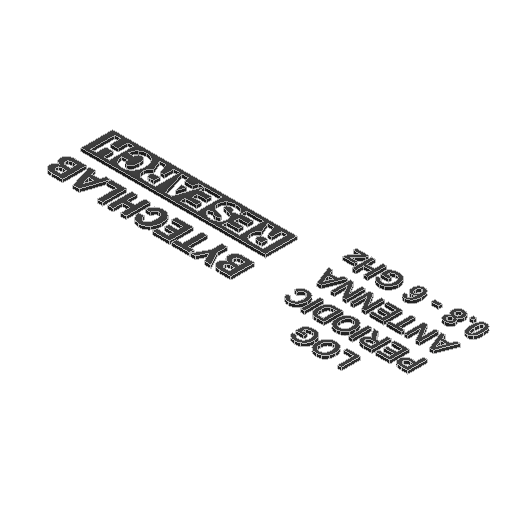
# Autodesk Inventor part: 3DP_PLA_Antenna_Case_Top_Logo_and_Name
Saved by Autodesk Inventor 2026.1 (Build 301233000, 233)
## iProperties
Created: 2025-11-20
Part Number: 3DP_PLA_Antenna_Case_Top_Logo_and_Name
Material: Generic
Document SubType Name: Modeling
Designer: User
Density: 1 g/cm^3
Appearance: Rubber - Black
Author: User
Autodesk Inventor part; units mm, degrees
(part 1 of 2)
ref_plane "YZ Plane" through (0, 0, 0) normal (1, 0, 0) x (0, 1, 0)
ref_plane "XZ Plane" through (0, 0, 0) normal (0, 1, 0) x (-1, 0, 0)
ref_plane "XY Plane" through (0, 0, 0) normal (0, 0, 1) x (1, 0, 0)
sketch "Sketch1" plane through (0, 0, 0) normal (0, 1, 0) x (-1, 0, 0)
  spline S0 degree 3 poles (1.4594, 11.82) (2.0835, 11.82) (2.5525, 11.7433) (2.8664, 11.59) knots 0 0 0 0 1 1 1 1
  line L0 (1.4594, 11.82) -> (2.0835, 11.82) construction
  line L1 (2.0835, 11.82) -> (2.5525, 11.7433) construction
  line L2 (2.5525, 11.7433) -> (2.8664, 11.59) construction
  spline S1 degree 3 poles (2.8664, 11.59) (3.1803, 11.4367) (3.4394, 11.2177) (3.6438, 10.933) knots 0 0 0 0 1 1 1 1
  line L3 (2.8664, 11.59) -> (3.1803, 11.4367) construction
  line L4 (3.1803, 11.4367) -> (3.4394, 11.2177) construction
  line L5 (3.4394, 11.2177) -> (3.6438, 10.933) construction
  spline S2 degree 3 poles (3.6438, 10.933) (3.8482, 10.6483) (3.9504, 10.3016) (3.9504, 9.8928) knots 0 0 0 0 1 1 1 1
  line L6 (3.6438, 10.933) -> (3.8482, 10.6483) construction
  line L7 (3.8482, 10.6483) -> (3.9504, 10.3016) construction
  line L8 (3.9504, 10.3016) -> (3.9504, 9.8928) construction
  spline S3 degree 3 poles (3.9504, 9.8928) (3.9504, 9.0643) (3.5015, 8.5113) (2.6036, 8.2339) knots 0 0 0 0 1 1 1 1
  line L9 (3.9504, 9.8928) -> (3.9504, 9.0643) construction
  line L10 (3.9504, 9.0643) -> (3.5015, 8.5113) construction
  line L11 (3.5015, 8.5113) -> (2.6036, 8.2339) construction
  spline S4 degree 3 poles (2.6036, 8.2339) (3.1219, 8.1171) (3.5106, 7.8854) (3.7698, 7.5386) knots 0 0 0 0 1 1 1 1
  line L12 (2.6036, 8.2339) -> (3.1219, 8.1171) construction
  line L13 (3.1219, 8.1171) -> (3.5106, 7.8854) construction
  line L14 (3.5106, 7.8854) -> (3.7698, 7.5386) construction
  spline S5 degree 3 poles (3.7698, 7.5386) (4.0289, 7.1919) (4.1585, 6.8141) (4.1585, 6.4053) knots 0 0 0 0 1 1 1 1
  line L15 (3.7698, 7.5386) -> (4.0289, 7.1919) construction
  line L16 (4.0289, 7.1919) -> (4.1585, 6.8141) construction
  line L17 (4.1585, 6.8141) -> (4.1585, 6.4053) construction
  spline S6 degree 3 poles (4.1585, 6.4053) (4.1585, 5.8469) (3.9468, 5.3633) (3.5234, 4.9545) knots 0 0 0 0 1 1 1 1
  line L18 (4.1585, 6.4053) -> (4.1585, 5.8469) construction
  line L19 (4.1585, 5.8469) -> (3.9468, 5.3633) construction
  line L20 (3.9468, 5.3633) -> (3.5234, 4.9545) construction
  spline S7 degree 3 poles (3.5234, 4.9545) (3.1, 4.5494) (2.412, 4.3468) (1.4594, 4.3468) knots 0 0 0 0 1 1 1 1
  line L21 (3.5234, 4.9545) -> (3.1, 4.5494) construction
  line L22 (3.1, 4.5494) -> (2.412, 4.3468) construction
  line L23 (2.412, 4.3468) -> (1.4594, 4.3468) construction
  line L24 (-2.0226, 11.82) -> (1.4594, 11.82)
  line L25 (1.4594, 4.3468) -> (-2.0226, 4.3468)
  line L26 (-2.0226, 4.3468) -> (-2.0226, 11.82)
  spline S8 degree 3 poles (1.0488, 8.8635) (1.5342, 8.8635) (1.839, 8.9584) (1.9631, 9.1482) knots 0 0 0 0 1 1 1 1
  line L27 (1.0488, 8.8635) -> (1.5342, 8.8635) construction
  line L28 (1.5342, 8.8635) -> (1.839, 8.9584) construction
  line L29 (1.839, 8.9584) -> (1.9631, 9.1482) construction
  spline S9 degree 3 poles (1.9631, 9.1482) (2.0908, 9.3417) (2.1547, 9.526) (2.1547, 9.7012) knots 0 0 0 0 1 1 1 1
  line L30 (1.9631, 9.1482) -> (2.0908, 9.3417) construction
  line L31 (2.0908, 9.3417) -> (2.1547, 9.526) construction
  line L32 (2.1547, 9.526) -> (2.1547, 9.7012) construction
  spline S10 degree 3 poles (2.1547, 9.7012) (2.1547, 9.891) (2.1017, 10.0534) (1.9959, 10.1885) knots 0 0 0 0 1 1 1 1
  line L33 (2.1547, 9.7012) -> (2.1547, 9.891) construction
  line L34 (2.1547, 9.891) -> (2.1017, 10.0534) construction
  line L35 (2.1017, 10.0534) -> (1.9959, 10.1885) construction
  spline S11 degree 3 poles (1.9959, 10.1885) (1.8937, 10.3272) (1.7806, 10.4129) (1.6565, 10.4458) knots 0 0 0 0 1 1 1 1
  line L36 (1.9959, 10.1885) -> (1.8937, 10.3272) construction
  line L37 (1.8937, 10.3272) -> (1.7806, 10.4129) construction
  line L38 (1.7806, 10.4129) -> (1.6565, 10.4458) construction
  spline S12 degree 3 poles (1.6565, 10.4458) (1.5324, 10.4823) (1.2878, 10.5005) (0.9228, 10.5005) knots 0 0 0 0 1 1 1 1
  line L39 (1.6565, 10.4458) -> (1.5324, 10.4823) construction
  line L40 (1.5324, 10.4823) -> (1.2878, 10.5005) construction
  line L41 (1.2878, 10.5005) -> (0.9228, 10.5005) construction
  line L42 (-0.2762, 10.5005) -> (-0.2762, 8.8635)
  line L43 (-0.2762, 8.8635) -> (1.0488, 8.8635)
  line L44 (0.9228, 10.5005) -> (-0.2762, 10.5005)
  spline S13 degree 3 poles (1.0707, 5.7319) (1.5305, 5.7319) (1.8554, 5.8122) (2.0452, 5.9728) knots 0 0 0 0 1 1 1 1
  line L45 (1.0707, 5.7319) -> (1.5305, 5.7319) construction
  line L46 (1.5305, 5.7319) -> (1.8554, 5.8122) construction
  line L47 (1.8554, 5.8122) -> (2.0452, 5.9728) construction
  spline S14 degree 3 poles (2.0452, 5.9728) (2.235, 6.1334) (2.3299, 6.3579) (2.3299, 6.6462) knots 0 0 0 0 1 1 1 1
  line L48 (2.0452, 5.9728) -> (2.235, 6.1334) construction
  line L49 (2.235, 6.1334) -> (2.3299, 6.3579) construction
  line L50 (2.3299, 6.3579) -> (2.3299, 6.6462) construction
  spline S15 degree 3 poles (2.3299, 6.6462) (2.3299, 6.8871) (2.2386, 7.0952) (2.0561, 7.2704) knots 0 0 0 0 1 1 1 1
  line L51 (2.3299, 6.6462) -> (2.3299, 6.8871) construction
  line L52 (2.3299, 6.8871) -> (2.2386, 7.0952) construction
  line L53 (2.2386, 7.0952) -> (2.0561, 7.2704) construction
  spline S16 degree 3 poles (2.0561, 7.2704) (1.8736, 7.4456) (1.5707, 7.5332) (1.1473, 7.5332) knots 0 0 0 0 1 1 1 1
  line L54 (2.0561, 7.2704) -> (1.8736, 7.4456) construction
  line L55 (1.8736, 7.4456) -> (1.5707, 7.5332) construction
  line L56 (1.5707, 7.5332) -> (1.1473, 7.5332) construction
  line L57 (-0.2762, 7.5332) -> (-0.2762, 5.7319)
  line L58 (-0.2762, 5.7319) -> (1.0707, 5.7319)
  line L59 (1.1473, 7.5332) -> (-0.2762, 7.5332)
  line L60 (10.5805, 11.82) -> (8.2318, 7.4948)
  line L61 (8.2318, 7.4948) -> (8.2318, 4.3468)
  line L62 (8.2318, 4.3468) -> (6.4798, 4.3468)
  line L63 (6.4798, 4.3468) -> (6.4798, 7.4948)
  line L64 (6.4798, 7.4948) -> (4.1311, 11.82)
  line L65 (4.1311, 11.82) -> (6.1623, 11.82)
  line L66 (6.1623, 11.82) -> (7.5912, 8.984)
  line L67 (7.5912, 8.984) -> (9.0092, 11.82)
  line L68 (9.0092, 11.82) -> (10.5805, 11.82)
  line L69 (16.2907, 11.82) -> (16.2907, 10.3418)
  line L70 (16.2907, 10.3418) -> (14.4402, 10.3418)
  line L71 (14.4402, 10.3418) -> (14.4402, 4.3468)
  line L72 (14.4402, 4.3468) -> (12.6664, 4.3468)
  line L73 (12.6664, 4.3468) -> (12.6664, 10.3418)
  line L74 (12.6664, 10.3418) -> (10.8049, 10.3418)
  line L75 (10.8049, 10.3418) -> (10.8049, 11.82)
  line L76 (10.8049, 11.82) -> (16.2907, 11.82)
  line L77 (22.3788, 10.3965) -> (18.8147, 10.3965)
  line L78 (18.8147, 10.3965) -> (18.8147, 8.8635)
  line L79 (18.8147, 8.8635) -> (21.6178, 8.8635)
  line L80 (21.6178, 8.8635) -> (21.6178, 7.4565)
  line L81 (21.6178, 7.4565) -> (18.8147, 7.4565)
  line L82 (18.8147, 7.4565) -> (18.8147, 5.825)
  line L83 (18.8147, 5.825) -> (22.3788, 5.825)
  line L84 (22.3788, 5.825) -> (22.3788, 4.3468)
  line L85 (22.3788, 4.3468) -> (17.0353, 4.3468)
  line L86 (17.0353, 4.3468) -> (17.0353, 11.82)
  line L87 (17.0353, 11.82) -> (22.3788, 11.82)
  line L88 (22.3788, 11.82) -> (22.3788, 10.3965)
  spline S17 degree 3 poles (27.6237, 8.9238) (27.5981, 9.9786) (27.1875, 10.506) (26.3919, 10.506) knots 0 0 0 0 1 1 1 1
  line L89 (27.6237, 8.9238) -> (27.5981, 9.9786) construction
  line L90 (27.5981, 9.9786) -> (27.1875, 10.506) construction
  line L91 (27.1875, 10.506) -> (26.3919, 10.506) construction
  spline S18 degree 3 poles (26.3919, 10.506) (25.4794, 10.506) (25.0231, 9.6939) (25.0231, 8.0697) knots 0 0 0 0 1 1 1 1
  line L92 (26.3919, 10.506) -> (25.4794, 10.506) construction
  line L93 (25.4794, 10.506) -> (25.0231, 9.6939) construction
  line L94 (25.0231, 9.6939) -> (25.0231, 8.0697) construction
  spline S19 degree 3 poles (25.0231, 8.0697) (25.0231, 7.1317) (25.1472, 6.4948) (25.3954, 6.159) knots 0 0 0 0 1 1 1 1
  line L95 (25.0231, 8.0697) -> (25.0231, 7.1317) construction
  line L96 (25.0231, 7.1317) -> (25.1472, 6.4948) construction
  line L97 (25.1472, 6.4948) -> (25.3954, 6.159) construction
  spline S20 degree 3 poles (25.3954, 6.159) (25.6436, 5.8268) (25.9904, 5.6608) (26.4357, 5.6608) knots 0 0 0 0 1 1 1 1
  line L98 (25.3954, 6.159) -> (25.6436, 5.8268) construction
  line L99 (25.6436, 5.8268) -> (25.9904, 5.6608) construction
  line L100 (25.9904, 5.6608) -> (26.4357, 5.6608) construction
  spline S21 degree 3 poles (26.4357, 5.6608) (27.1583, 5.6608) (27.6, 6.1316) (27.7606, 7.0733) knots 0 0 0 0 1 1 1 1
  line L101 (26.4357, 5.6608) -> (27.1583, 5.6608) construction
  line L102 (27.1583, 5.6608) -> (27.6, 6.1316) construction
  line L103 (27.6, 6.1316) -> (27.7606, 7.0733) construction
  line L104 (29.4578, 9.0387) -> (27.6237, 8.9238)
  spline S22 degree 3 poles (29.4578, 6.9692) (29.3483, 6.075) (29.0143, 5.3943) (28.4559, 4.9271) knots 0 0 0 0 1 1 1 1
  line L105 (29.4578, 6.9692) -> (29.3483, 6.075) construction
  line L106 (29.3483, 6.075) -> (29.0143, 5.3943) construction
  line L107 (29.0143, 5.3943) -> (28.4559, 4.9271) construction
  spline S23 degree 3 poles (28.4559, 4.9271) (27.9011, 4.4636) (27.2204, 4.2318) (26.4138, 4.2318) knots 0 0 0 0 1 1 1 1
  line L108 (28.4559, 4.9271) -> (27.9011, 4.4636) construction
  line L109 (27.9011, 4.4636) -> (27.2204, 4.2318) construction
  line L110 (27.2204, 4.2318) -> (26.4138, 4.2318) construction
  spline S24 degree 3 poles (26.4138, 4.2318) (25.4246, 4.2318) (24.6198, 4.5731) (23.9993, 5.2556) knots 0 0 0 0 1 1 1 1
  line L111 (26.4138, 4.2318) -> (25.4246, 4.2318) construction
  line L112 (25.4246, 4.2318) -> (24.6198, 4.5731) construction
  line L113 (24.6198, 4.5731) -> (23.9993, 5.2556) construction
  spline S25 degree 3 poles (23.9993, 5.2556) (23.3825, 5.9381) (23.0741, 6.8816) (23.0741, 8.0861) knots 0 0 0 0 1 1 1 1
  line L114 (23.9993, 5.2556) -> (23.3825, 5.9381) construction
  line L115 (23.3825, 5.9381) -> (23.0741, 6.8816) construction
  line L116 (23.0741, 6.8816) -> (23.0741, 8.0861) construction
  spline S26 degree 3 poles (23.0741, 8.0861) (23.0741, 9.2139) (23.3734, 10.1374) (23.972, 10.8564) knots 0 0 0 0 1 1 1 1
  line L117 (23.0741, 8.0861) -> (23.0741, 9.2139) construction
  line L118 (23.0741, 9.2139) -> (23.3734, 10.1374) construction
  line L119 (23.3734, 10.1374) -> (23.972, 10.8564) construction
  spline S27 degree 3 poles (23.972, 10.8564) (24.5706, 11.5754) (25.3881, 11.9349) (26.4247, 11.9349) knots 0 0 0 0 1 1 1 1
  line L120 (23.972, 10.8564) -> (24.5706, 11.5754) construction
  line L121 (24.5706, 11.5754) -> (25.3881, 11.9349) construction
  line L122 (25.3881, 11.9349) -> (26.4247, 11.9349) construction
  spline S28 degree 3 poles (26.4247, 11.9349) (28.2205, 11.9349) (29.2315, 10.9695) (29.4578, 9.0387) knots 0 0 0 0 1 1 1 1
  line L123 (26.4247, 11.9349) -> (28.2205, 11.9349) construction
  line L124 (28.2205, 11.9349) -> (29.2315, 10.9695) construction
  line L125 (29.2315, 10.9695) -> (29.4578, 9.0387) construction
  line L126 (27.7606, 7.0733) -> (29.4578, 6.9692)
  line L127 (36.2411, 11.82) -> (36.2411, 4.3468)
  line L128 (36.2411, 4.3468) -> (34.522, 4.3468)
  line L129 (34.522, 4.3468) -> (34.522, 7.4291)
  line L130 (34.522, 7.4291) -> (32.1843, 7.4291)
  line L131 (32.1843, 7.4291) -> (32.1843, 4.3468)
  line L132 (32.1843, 4.3468) -> (30.4651, 4.3468)
  line L133 (30.4651, 4.3468) -> (30.4651, 11.82)
  line L134 (30.4651, 11.82) -> (32.1843, 11.82)
  line L135 (32.1843, 11.82) -> (32.1843, 8.9073)
  line L136 (32.1843, 8.9073) -> (34.522, 8.9073)
  line L137 (34.522, 8.9073) -> (34.522, 11.82)
  line L138 (34.522, 11.82) -> (36.2411, 11.82)
  line L139 (39.5096, 5.825) -> (42.4824, 5.825)
  line L140 (42.4824, 5.825) -> (42.4824, 4.3468)
  line L141 (42.4824, 4.3468) -> (37.7358, 4.3468)
  line L142 (37.7358, 4.3468) -> (37.7358, 11.82)
  line L143 (37.7358, 11.82) -> (39.5096, 11.82)
  line L144 (39.5096, 11.82) -> (39.5096, 5.825)
  line L145 (47.054, 11.82) -> (49.3917, 4.3468)
  line L146 (49.3917, 4.3468) -> (47.5084, 4.3468)
  line L147 (47.5084, 4.3468) -> (47.054, 5.8852)
  line L148 (47.054, 5.8852) -> (44.6341, 5.8852)
  line L149 (44.6341, 5.8852) -> (44.1632, 4.3468)
  line L150 (44.1632, 4.3468) -> (42.6303, 4.3468)
  line L151 (42.6303, 4.3468) -> (45.0228, 11.82)
  line L152 (45.0228, 11.82) -> (47.054, 11.82)
  line L153 (45.0556, 7.2649) -> (46.6433, 7.2649)
  line L154 (46.6433, 7.2649) -> (45.8495, 9.8873)
  line L155 (45.8495, 9.8873) -> (45.0556, 7.2649)
  spline S29 degree 3 poles (53.6785, 11.82) (54.3027, 11.82) (54.7717, 11.7433) (55.0856, 11.59) knots 0 0 0 0 1 1 1 1
  line L156 (53.6785, 11.82) -> (54.3027, 11.82) construction
  line L157 (54.3027, 11.82) -> (54.7717, 11.7433) construction
  line L158 (54.7717, 11.7433) -> (55.0856, 11.59) construction
  spline S30 degree 3 poles (55.0856, 11.59) (55.3995, 11.4367) (55.6586, 11.2177) (55.863, 10.933) knots 0 0 0 0 1 1 1 1
  line L159 (55.0856, 11.59) -> (55.3995, 11.4367) construction
  line L160 (55.3995, 11.4367) -> (55.6586, 11.2177) construction
  line L161 (55.6586, 11.2177) -> (55.863, 10.933) construction
  spline S31 degree 3 poles (55.863, 10.933) (56.0674, 10.6483) (56.1696, 10.3016) (56.1696, 9.8928) knots 0 0 0 0 1 1 1 1
  line L162 (55.863, 10.933) -> (56.0674, 10.6483) construction
  line L163 (56.0674, 10.6483) -> (56.1696, 10.3016) construction
  line L164 (56.1696, 10.3016) -> (56.1696, 9.8928) construction
  spline S32 degree 3 poles (56.1696, 9.8928) (56.1696, 9.0643) (55.7206, 8.5113) (54.8228, 8.2339) knots 0 0 0 0 1 1 1 1
  line L165 (56.1696, 9.8928) -> (56.1696, 9.0643) construction
  line L166 (56.1696, 9.0643) -> (55.7206, 8.5113) construction
  line L167 (55.7206, 8.5113) -> (54.8228, 8.2339) construction
  spline S33 degree 3 poles (54.8228, 8.2339) (55.3411, 8.1171) (55.7298, 7.8854) (55.9889, 7.5386) knots 0 0 0 0 1 1 1 1
  line L168 (54.8228, 8.2339) -> (55.3411, 8.1171) construction
  line L169 (55.3411, 8.1171) -> (55.7298, 7.8854) construction
  line L170 (55.7298, 7.8854) -> (55.9889, 7.5386) construction
  spline S34 degree 3 poles (55.9889, 7.5386) (56.2481, 7.1919) (56.3776, 6.8141) (56.3776, 6.4053) knots 0 0 0 0 1 1 1 1
  line L171 (55.9889, 7.5386) -> (56.2481, 7.1919) construction
  line L172 (56.2481, 7.1919) -> (56.3776, 6.8141) construction
  line L173 (56.3776, 6.8141) -> (56.3776, 6.4053) construction
  spline S35 degree 3 poles (56.3776, 6.4053) (56.3776, 5.8469) (56.1659, 5.3633) (55.7425, 4.9545) knots 0 0 0 0 1 1 1 1
  line L174 (56.3776, 6.4053) -> (56.3776, 5.8469) construction
  line L175 (56.3776, 5.8469) -> (56.1659, 5.3633) construction
  line L176 (56.1659, 5.3633) -> (55.7425, 4.9545) construction
  spline S36 degree 3 poles (55.7425, 4.9545) (55.3192, 4.5494) (54.6312, 4.3468) (53.6785, 4.3468) knots 0 0 0 0 1 1 1 1
  line L177 (55.7425, 4.9545) -> (55.3192, 4.5494) construction
  line L178 (55.3192, 4.5494) -> (54.6312, 4.3468) construction
  line L179 (54.6312, 4.3468) -> (53.6785, 4.3468) construction
  line L180 (50.1965, 11.82) -> (53.6785, 11.82)
  line L181 (53.6785, 4.3468) -> (50.1965, 4.3468)
  line L182 (50.1965, 4.3468) -> (50.1965, 11.82)
  spline S37 degree 3 poles (53.2679, 8.8635) (53.7534, 8.8635) (54.0581, 8.9584) (54.1822, 9.1482) knots 0 0 0 0 1 1 1 1
  line L183 (53.2679, 8.8635) -> (53.7534, 8.8635) construction
  line L184 (53.7534, 8.8635) -> (54.0581, 8.9584) construction
  line L185 (54.0581, 8.9584) -> (54.1822, 9.1482) construction
  spline S38 degree 3 poles (54.1822, 9.1482) (54.31, 9.3417) (54.3738, 9.526) (54.3738, 9.7012) knots 0 0 0 0 1 1 1 1
  line L186 (54.1822, 9.1482) -> (54.31, 9.3417) construction
  line L187 (54.31, 9.3417) -> (54.3738, 9.526) construction
  line L188 (54.3738, 9.526) -> (54.3738, 9.7012) construction
  spline S39 degree 3 poles (54.3738, 9.7012) (54.3738, 9.891) (54.3209, 10.0534) (54.2151, 10.1885) knots 0 0 0 0 1 1 1 1
  line L189 (54.3738, 9.7012) -> (54.3738, 9.891) construction
  line L190 (54.3738, 9.891) -> (54.3209, 10.0534) construction
  line L191 (54.3209, 10.0534) -> (54.2151, 10.1885) construction
  spline S40 degree 3 poles (54.2151, 10.1885) (54.1129, 10.3272) (53.9997, 10.4129) (53.8756, 10.4458) knots 0 0 0 0 1 1 1 1
  line L192 (54.2151, 10.1885) -> (54.1129, 10.3272) construction
  line L193 (54.1129, 10.3272) -> (53.9997, 10.4129) construction
  line L194 (53.9997, 10.4129) -> (53.8756, 10.4458) construction
  spline S41 degree 3 poles (53.8756, 10.4458) (53.7515, 10.4823) (53.507, 10.5005) (53.142, 10.5005) knots 0 0 0 0 1 1 1 1
  line L195 (53.8756, 10.4458) -> (53.7515, 10.4823) construction
  line L196 (53.7515, 10.4823) -> (53.507, 10.5005) construction
  line L197 (53.507, 10.5005) -> (53.142, 10.5005) construction
  line L198 (51.943, 10.5005) -> (51.943, 8.8635)
  line L199 (51.943, 8.8635) -> (53.2679, 8.8635)
  line L200 (53.142, 10.5005) -> (51.943, 10.5005)
  spline S42 degree 3 poles (53.2898, 5.7319) (53.7497, 5.7319) (54.0745, 5.8122) (54.2643, 5.9728) knots 0 0 0 0 1 1 1 1
  line L201 (53.2898, 5.7319) -> (53.7497, 5.7319) construction
  line L202 (53.7497, 5.7319) -> (54.0745, 5.8122) construction
  line L203 (54.0745, 5.8122) -> (54.2643, 5.9728) construction
  spline S43 degree 3 poles (54.2643, 5.9728) (54.4541, 6.1334) (54.549, 6.3579) (54.549, 6.6462) knots 0 0 0 0 1 1 1 1
  line L204 (54.2643, 5.9728) -> (54.4541, 6.1334) construction
  line L205 (54.4541, 6.1334) -> (54.549, 6.3579) construction
  line L206 (54.549, 6.3579) -> (54.549, 6.6462) construction
  spline S44 degree 3 poles (54.549, 6.6462) (54.549, 6.8871) (54.4578, 7.0952) (54.2753, 7.2704) knots 0 0 0 0 1 1 1 1
  line L207 (54.549, 6.6462) -> (54.549, 6.8871) construction
  line L208 (54.549, 6.8871) -> (54.4578, 7.0952) construction
  line L209 (54.4578, 7.0952) -> (54.2753, 7.2704) construction
  spline S45 degree 3 poles (54.2753, 7.2704) (54.0928, 7.4456) (53.7898, 7.5332) (53.3665, 7.5332) knots 0 0 0 0 1 1 1 1
  line L210 (54.2753, 7.2704) -> (54.0928, 7.4456) construction
  line L211 (54.0928, 7.4456) -> (53.7898, 7.5332) construction
  line L212 (53.7898, 7.5332) -> (53.3665, 7.5332) construction
  line L213 (51.943, 7.5332) -> (51.943, 5.7319)
  line L214 (51.943, 5.7319) -> (53.2898, 5.7319)
  line L215 (53.3665, 7.5332) -> (51.943, 7.5332)
  line L216 (-1.4592, 0.5085) -> (55.8142, 0.5085)
  line L217 (55.8142, 0.5085) -> (55.8142, -9.3243)
  line L218 (55.8142, -9.3243) -> (-1.4592, -9.3243)
  line L219 (-1.4592, -9.3243) -> (-1.4592, 0.5085)
  spline S46 degree 3 poles (3.7095, -0.6713) (4.3154, -0.6713) (4.8009, -0.7425) (5.1658, -0.8848) knots 0 0 0 0 1 1 1 1
  line L220 (3.7095, -0.6713) -> (4.3154, -0.6713) construction
  line L221 (4.3154, -0.6713) -> (4.8009, -0.7425) construction
  line L222 (4.8009, -0.7425) -> (5.1658, -0.8848) construction
  spline S47 degree 3 poles (5.1658, -0.8848) (5.5345, -1.0235) (5.8393, -1.2808) (6.0801, -1.6568) knots 0 0 0 0 1 1 1 1
  line L223 (5.1658, -0.8848) -> (5.5345, -1.0235) construction
  line L224 (5.5345, -1.0235) -> (5.8393, -1.2808) construction
  line L225 (5.8393, -1.2808) -> (6.0801, -1.6568) construction
  spline S48 degree 3 poles (6.0801, -1.6568) (6.321, -2.0327) (6.4415, -2.4506) (6.4415, -2.9105) knots 0 0 0 0 1 1 1 1
  line L226 (6.0801, -1.6568) -> (6.321, -2.0327) construction
  line L227 (6.321, -2.0327) -> (6.4415, -2.4506) construction
  line L228 (6.4415, -2.4506) -> (6.4415, -2.9105) construction
  spline S49 degree 3 poles (6.4415, -2.9105) (6.4415, -3.8084) (6.009, -4.4526) (5.1439, -4.8431) knots 0 0 0 0 1 1 1 1
  line L229 (6.4415, -2.9105) -> (6.4415, -3.8084) construction
  line L230 (6.4415, -3.8084) -> (6.009, -4.4526) construction
  line L231 (6.009, -4.4526) -> (5.1439, -4.8431) construction
  line L232 (2.1875, -5.1826) -> (2.1875, -8.1445)
  line L233 (2.1875, -8.1445) -> (0.4246, -8.1445)
  line L234 (0.4246, -8.1445) -> (0.4246, -0.6713)
  line L235 (0.4246, -0.6713) -> (3.7095, -0.6713)
  line L236 (5.1439, -4.8431) -> (6.5236, -8.1445)
  line L237 (6.5236, -8.1445) -> (4.591, -8.1445)
  line L238 (4.591, -8.1445) -> (3.4413, -5.1826)
  line L239 (3.4413, -5.1826) -> (2.1875, -5.1826)
  spline S50 degree 3 poles (3.2606, -3.9069) (3.611, -3.9069) (3.8647, -3.8832) (4.0216, -3.8358) knots 0 0 0 0 1 1 1 1
  line L240 (3.2606, -3.9069) -> (3.611, -3.9069) construction
  line L241 (3.611, -3.9069) -> (3.8647, -3.8832) construction
  line L242 (3.8647, -3.8832) -> (4.0216, -3.8358) construction
  spline S51 degree 3 poles (4.0216, -3.8358) (4.1822, -3.7847) (4.3245, -3.6752) (4.4486, -3.5073) knots 0 0 0 0 1 1 1 1
  line L243 (4.0216, -3.8358) -> (4.1822, -3.7847) construction
  line L244 (4.1822, -3.7847) -> (4.3245, -3.6752) construction
  line L245 (4.3245, -3.6752) -> (4.4486, -3.5073) construction
  spline S52 degree 3 poles (4.4486, -3.5073) (4.5727, -3.3357) (4.6348, -3.1405) (4.6348, -2.9215) knots 0 0 0 0 1 1 1 1
  line L246 (4.4486, -3.5073) -> (4.5727, -3.3357) construction
  line L247 (4.5727, -3.3357) -> (4.6348, -3.1405) construction
  line L248 (4.6348, -3.1405) -> (4.6348, -2.9215) construction
  spline S53 degree 3 poles (4.6348, -2.9215) (4.6348, -2.7134) (4.5727, -2.5273) (4.4486, -2.363) knots 0 0 0 0 1 1 1 1
  line L249 (4.6348, -2.9215) -> (4.6348, -2.7134) construction
  line L250 (4.6348, -2.7134) -> (4.5727, -2.5273) construction
  line L251 (4.5727, -2.5273) -> (4.4486, -2.363) construction
  spline S54 degree 3 poles (4.4486, -2.363) (4.3245, -2.1988) (4.1895, -2.0984) (4.0435, -2.0619) knots 0 0 0 0 1 1 1 1
  line L252 (4.4486, -2.363) -> (4.3245, -2.1988) construction
  line L253 (4.3245, -2.1988) -> (4.1895, -2.0984) construction
  line L254 (4.1895, -2.0984) -> (4.0435, -2.0619) construction
  spline S55 degree 3 poles (4.0435, -2.0619) (3.8975, -2.0218) (3.6238, -2.0017) (3.2223, -2.0017) knots 0 0 0 0 1 1 1 1
  line L255 (4.0435, -2.0619) -> (3.8975, -2.0218) construction
  line L256 (3.8975, -2.0218) -> (3.6238, -2.0017) construction
  line L257 (3.6238, -2.0017) -> (3.2223, -2.0017) construction
  line L258 (2.1875, -2.0017) -> (2.1875, -3.9069)
  line L259 (2.1875, -3.9069) -> (3.2606, -3.9069)
  line L260 (3.2223, -2.0017) -> (2.1875, -2.0017)
  line L261 (13.1318, -2.0948) -> (9.5676, -2.0948)
  line L262 (9.5676, -2.0948) -> (9.5676, -3.6277)
  line L263 (9.5676, -3.6277) -> (12.3708, -3.6277)
  line L264 (12.3708, -3.6277) -> (12.3708, -5.0348)
  line L265 (12.3708, -5.0348) -> (9.5676, -5.0348)
  line L266 (9.5676, -5.0348) -> (9.5676, -6.6663)
  line L267 (9.5676, -6.6663) -> (13.1318, -6.6663)
  line L268 (13.1318, -6.6663) -> (13.1318, -8.1445)
  line L269 (13.1318, -8.1445) -> (7.7883, -8.1445)
  line L270 (7.7883, -8.1445) -> (7.7883, -0.6713)
  line L271 (7.7883, -0.6713) -> (13.1318, -0.6713)
  line L272 (13.1318, -0.6713) -> (13.1318, -2.0948)
  spline S56 degree 3 poles (17.8566, -2.812) (17.6558, -2.2207) (17.2306, -1.925) (16.5809, -1.925) knots 0 0 0 0 1 1 1 1
  line L273 (17.8566, -2.812) -> (17.6558, -2.2207) construction
  line L274 (17.6558, -2.2207) -> (17.2306, -1.925) construction
  line L275 (17.2306, -1.925) -> (16.5809, -1.925) construction
  spline S57 degree 3 poles (16.5809, -1.925) (15.8874, -1.925) (15.5407, -2.1495) (15.5407, -2.5984) knots 0 0 0 0 1 1 1 1
  line L276 (16.5809, -1.925) -> (15.8874, -1.925) construction
  line L277 (15.8874, -1.925) -> (15.5407, -2.1495) construction
  line L278 (15.5407, -2.1495) -> (15.5407, -2.5984) construction
  spline S58 degree 3 poles (15.5407, -2.5984) (15.5407, -2.7773) (15.6046, -2.9288) (15.7323, -3.0529) knots 0 0 0 0 1 1 1 1
  line L279 (15.5407, -2.5984) -> (15.5407, -2.7773) construction
  line L280 (15.5407, -2.7773) -> (15.6046, -2.9288) construction
  line L281 (15.6046, -2.9288) -> (15.7323, -3.0529) construction
  spline S59 degree 3 poles (15.7323, -3.0529) (15.8637, -3.177) (16.1575, -3.2846) (16.6138, -3.3759) knots 0 0 0 0 1 1 1 1
  line L282 (15.7323, -3.0529) -> (15.8637, -3.177) construction
  line L283 (15.8637, -3.177) -> (16.1575, -3.2846) construction
  line L284 (16.1575, -3.2846) -> (16.6138, -3.3759) construction
  spline S60 degree 3 poles (16.6138, -3.3759) (17.3766, -3.5292) (17.935, -3.6843) (18.2891, -3.8412) knots 0 0 0 0 1 1 1 1
  line L285 (16.6138, -3.3759) -> (17.3766, -3.5292) construction
  line L286 (17.3766, -3.5292) -> (17.935, -3.6843) construction
  line L287 (17.935, -3.6843) -> (18.2891, -3.8412) construction
  spline S61 degree 3 poles (18.2891, -3.8412) (18.6431, -3.9982) (18.9406, -4.2518) (19.1815, -4.6022) knots 0 0 0 0 1 1 1 1
  line L288 (18.2891, -3.8412) -> (18.6431, -3.9982) construction
  line L289 (18.6431, -3.9982) -> (18.9406, -4.2518) construction
  line L290 (18.9406, -4.2518) -> (19.1815, -4.6022) construction
  spline S62 degree 3 poles (19.1815, -4.6022) (19.426, -4.949) (19.5483, -5.3377) (19.5483, -5.7684) knots 0 0 0 0 1 1 1 1
  line L291 (19.1815, -4.6022) -> (19.426, -4.949) construction
  line L292 (19.426, -4.949) -> (19.5483, -5.3377) construction
  line L293 (19.5483, -5.3377) -> (19.5483, -5.7684) construction
  spline S63 degree 3 poles (19.5483, -5.7684) (19.5483, -6.4436) (19.2873, -7.0276) (18.7654, -7.5203) knots 0 0 0 0 1 1 1 1
  line L294 (19.5483, -5.7684) -> (19.5483, -6.4436) construction
  line L295 (19.5483, -6.4436) -> (19.2873, -7.0276) construction
  line L296 (19.2873, -7.0276) -> (18.7654, -7.5203) construction
  spline S64 degree 3 poles (18.7654, -7.5203) (18.2471, -8.0131) (17.477, -8.2594) (16.455, -8.2594) knots 0 0 0 0 1 1 1 1
  line L297 (18.7654, -7.5203) -> (18.2471, -8.0131) construction
  line L298 (18.2471, -8.0131) -> (17.477, -8.2594) construction
  line L299 (17.477, -8.2594) -> (16.455, -8.2594) construction
  spline S65 degree 3 poles (16.455, -8.2594) (15.6885, -8.2594) (15.0352, -8.0861) (14.495, -7.7393) knots 0 0 0 0 1 1 1 1
  line L300 (16.455, -8.2594) -> (15.6885, -8.2594) construction
  line L301 (15.6885, -8.2594) -> (15.0352, -8.0861) construction
  line L302 (15.0352, -8.0861) -> (14.495, -7.7393) construction
  spline S66 degree 3 poles (14.495, -7.7393) (13.9585, -7.3889) (13.6044, -6.8707) (13.4329, -6.1845) knots 0 0 0 0 1 1 1 1
  line L303 (14.495, -7.7393) -> (13.9585, -7.3889) construction
  line L304 (13.9585, -7.3889) -> (13.6044, -6.8707) construction
  line L305 (13.6044, -6.8707) -> (13.4329, -6.1845) construction
  line L306 (19.3457, -2.3137) -> (17.8566, -2.812)
  spline S67 degree 3 poles (15.0534, -5.8177) (15.2359, -6.5148) (15.7433, -6.8634) (16.5754, -6.8634) knots 0 0 0 0 1 1 1 1
  line L307 (15.0534, -5.8177) -> (15.2359, -6.5148) construction
  line L308 (15.2359, -6.5148) -> (15.7433, -6.8634) construction
  line L309 (15.7433, -6.8634) -> (16.5754, -6.8634) construction
  spline S68 degree 3 poles (16.5754, -6.8634) (16.9769, -6.8634) (17.2762, -6.7867) (17.4733, -6.6334) knots 0 0 0 0 1 1 1 1
  line L310 (16.5754, -6.8634) -> (16.9769, -6.8634) construction
  line L311 (16.9769, -6.8634) -> (17.2762, -6.7867) construction
  line L312 (17.2762, -6.7867) -> (17.4733, -6.6334) construction
  spline S69 degree 3 poles (17.4733, -6.6334) (17.6704, -6.4765) (17.769, -6.2903) (17.769, -6.075) knots 0 0 0 0 1 1 1 1
  line L313 (17.4733, -6.6334) -> (17.6704, -6.4765) construction
  line L314 (17.6704, -6.4765) -> (17.769, -6.2903) construction
  line L315 (17.769, -6.2903) -> (17.769, -6.075) construction
  spline S70 degree 3 poles (17.769, -6.075) (17.769, -5.856) (17.6795, -5.6863) (17.5007, -5.5658) knots 0 0 0 0 1 1 1 1
  line L316 (17.769, -6.075) -> (17.769, -5.856) construction
  line L317 (17.769, -5.856) -> (17.6795, -5.6863) construction
  line L318 (17.6795, -5.6863) -> (17.5007, -5.5658) construction
  spline S71 degree 3 poles (17.5007, -5.5658) (17.3218, -5.4454) (16.9769, -5.3322) (16.4659, -5.2264) knots 0 0 0 0 1 1 1 1
  line L319 (17.5007, -5.5658) -> (17.3218, -5.4454) construction
  line L320 (17.3218, -5.4454) -> (16.9769, -5.3322) construction
  line L321 (16.9769, -5.3322) -> (16.4659, -5.2264) construction
  spline S72 degree 3 poles (16.4659, -5.2264) (15.5133, -5.0293) (14.8344, -4.761) (14.4293, -4.4216) knots 0 0 0 0 1 1 1 1
  line L322 (16.4659, -5.2264) -> (15.5133, -5.0293) construction
  line L323 (15.5133, -5.0293) -> (14.8344, -4.761) construction
  line L324 (14.8344, -4.761) -> (14.4293, -4.4216) construction
  spline S73 degree 3 poles (14.4293, -4.4216) (14.0242, -4.0785) (13.8216, -3.5784) (13.8216, -2.9215) knots 0 0 0 0 1 1 1 1
  line L325 (14.4293, -4.4216) -> (14.0242, -4.0785) construction
  line L326 (14.0242, -4.0785) -> (13.8216, -3.5784) construction
  line L327 (13.8216, -3.5784) -> (13.8216, -2.9215) construction
  spline S74 degree 3 poles (13.8216, -2.9215) (13.8216, -2.2572) (14.0625, -1.6969) (14.5443, -1.2407) knots 0 0 0 0 1 1 1 1
  line L328 (13.8216, -2.9215) -> (13.8216, -2.2572) construction
  line L329 (13.8216, -2.2572) -> (14.0625, -1.6969) construction
  line L330 (14.0625, -1.6969) -> (14.5443, -1.2407) construction
  spline S75 degree 3 poles (14.5443, -1.2407) (15.0297, -0.7844) (15.6867, -0.5563) (16.5152, -0.5563) knots 0 0 0 0 1 1 1 1
  line L331 (14.5443, -1.2407) -> (15.0297, -0.7844) construction
  line L332 (15.0297, -0.7844) -> (15.6867, -0.5563) construction
  line L333 (15.6867, -0.5563) -> (16.5152, -0.5563) construction
  spline S76 degree 3 poles (16.5152, -0.5563) (17.9825, -0.5563) (18.926, -1.1421) (19.3457, -2.3137) knots 0 0 0 0 1 1 1 1
  line L334 (16.5152, -0.5563) -> (17.9825, -0.5563) construction
  line L335 (17.9825, -0.5563) -> (18.926, -1.1421) construction
  line L336 (18.926, -1.1421) -> (19.3457, -2.3137) construction
  line L337 (13.4329, -6.1845) -> (15.0534, -5.8177)
  line L338 (26.0305, -2.0948) -> (22.4664, -2.0948)
  line L339 (22.4664, -2.0948) -> (22.4664, -3.6277)
  line L340 (22.4664, -3.6277) -> (25.2695, -3.6277)
  line L341 (25.2695, -3.6277) -> (25.2695, -5.0348)
  line L342 (25.2695, -5.0348) -> (22.4664, -5.0348)
  line L343 (22.4664, -5.0348) -> (22.4664, -6.6663)
  line L344 (22.4664, -6.6663) -> (26.0305, -6.6663)
  line L345 (26.0305, -6.6663) -> (26.0305, -8.1445)
  line L346 (26.0305, -8.1445) -> (20.6871, -8.1445)
  line L347 (20.6871, -8.1445) -> (20.6871, -0.6713)
  line L348 (20.6871, -0.6713) -> (26.0305, -0.6713)
  line L349 (26.0305, -0.6713) -> (26.0305, -2.0948)
  line L350 (30.7553, -0.6713) -> (33.0931, -8.1445)
  line L351 (33.0931, -8.1445) -> (31.2097, -8.1445)
  line L352 (31.2097, -8.1445) -> (30.7553, -6.606)
  line L353 (30.7553, -6.606) -> (28.3354, -6.606)
  line L354 (28.3354, -6.606) -> (27.8646, -8.1445)
  line L355 (27.8646, -8.1445) -> (26.3316, -8.1445)
  line L356 (26.3316, -8.1445) -> (28.7241, -0.6713)
  line L357 (28.7241, -0.6713) -> (30.7553, -0.6713)
  line L358 (28.757, -5.2264) -> (30.3447, -5.2264)
  line L359 (30.3447, -5.2264) -> (29.5508, -2.6039)
  line L360 (29.5508, -2.6039) -> (28.757, -5.2264)
  spline S77 degree 3 poles (37.1828, -0.6713) (37.7887, -0.6713) (38.2741, -0.7425) (38.6391, -0.8848) knots 0 0 0 0 1 1 1 1
  line L361 (37.1828, -0.6713) -> (37.7887, -0.6713) construction
  line L362 (37.7887, -0.6713) -> (38.2741, -0.7425) construction
  line L363 (38.2741, -0.7425) -> (38.6391, -0.8848) construction
  spline S78 degree 3 poles (38.6391, -0.8848) (39.0077, -1.0235) (39.3125, -1.2808) (39.5534, -1.6568) knots 0 0 0 0 1 1 1 1
  line L364 (38.6391, -0.8848) -> (39.0077, -1.0235) construction
  line L365 (39.0077, -1.0235) -> (39.3125, -1.2808) construction
  line L366 (39.3125, -1.2808) -> (39.5534, -1.6568) construction
  spline S79 degree 3 poles (39.5534, -1.6568) (39.7943, -2.0327) (39.9147, -2.4506) (39.9147, -2.9105) knots 0 0 0 0 1 1 1 1
  line L367 (39.5534, -1.6568) -> (39.7943, -2.0327) construction
  line L368 (39.7943, -2.0327) -> (39.9147, -2.4506) construction
  line L369 (39.9147, -2.4506) -> (39.9147, -2.9105) construction
  spline S80 degree 3 poles (39.9147, -2.9105) (39.9147, -3.8084) (39.4822, -4.4526) (38.6172, -4.8431) knots 0 0 0 0 1 1 1 1
  line L370 (39.9147, -2.9105) -> (39.9147, -3.8084) construction
  line L371 (39.9147, -3.8084) -> (39.4822, -4.4526) construction
  line L372 (39.4822, -4.4526) -> (38.6172, -4.8431) construction
  line L373 (35.6608, -5.1826) -> (35.6608, -8.1445)
  line L374 (35.6608, -8.1445) -> (33.8979, -8.1445)
  line L375 (33.8979, -8.1445) -> (33.8979, -0.6713)
  line L376 (33.8979, -0.6713) -> (37.1828, -0.6713)
  line L377 (38.6172, -4.8431) -> (39.9969, -8.1445)
  line L378 (39.9969, -8.1445) -> (38.0642, -8.1445)
  line L379 (38.0642, -8.1445) -> (36.9145, -5.1826)
  line L380 (36.9145, -5.1826) -> (35.6608, -5.1826)
  spline S81 degree 3 poles (36.7339, -3.9069) (37.0842, -3.9069) (37.3379, -3.8832) (37.4949, -3.8358) knots 0 0 0 0 1 1 1 1
  line L381 (36.7339, -3.9069) -> (37.0842, -3.9069) construction
  line L382 (37.0842, -3.9069) -> (37.3379, -3.8832) construction
  line L383 (37.3379, -3.8832) -> (37.4949, -3.8358) construction
  spline S82 degree 3 poles (37.4949, -3.8358) (37.6555, -3.7847) (37.7978, -3.6752) (37.9219, -3.5073) knots 0 0 0 0 1 1 1 1
  line L384 (37.4949, -3.8358) -> (37.6555, -3.7847) construction
  line L385 (37.6555, -3.7847) -> (37.7978, -3.6752) construction
  line L386 (37.7978, -3.6752) -> (37.9219, -3.5073) construction
  spline S83 degree 3 poles (37.9219, -3.5073) (38.046, -3.3357) (38.108, -3.1405) (38.108, -2.9215) knots 0 0 0 0 1 1 1 1
  line L387 (37.9219, -3.5073) -> (38.046, -3.3357) construction
  line L388 (38.046, -3.3357) -> (38.108, -3.1405) construction
  line L389 (38.108, -3.1405) -> (38.108, -2.9215) construction
  spline S84 degree 3 poles (38.108, -2.9215) (38.108, -2.7134) (38.046, -2.5273) (37.9219, -2.363) knots 0 0 0 0 1 1 1 1
  line L390 (38.108, -2.9215) -> (38.108, -2.7134) construction
  line L391 (38.108, -2.7134) -> (38.046, -2.5273) construction
  line L392 (38.046, -2.5273) -> (37.9219, -2.363) construction
  spline S85 degree 3 poles (37.9219, -2.363) (37.7978, -2.1988) (37.6628, -2.0984) (37.5168, -2.0619) knots 0 0 0 0 1 1 1 1
  line L393 (37.9219, -2.363) -> (37.7978, -2.1988) construction
  line L394 (37.7978, -2.1988) -> (37.6628, -2.0984) construction
  line L395 (37.6628, -2.0984) -> (37.5168, -2.0619) construction
  spline S86 degree 3 poles (37.5168, -2.0619) (37.3708, -2.0218) (37.097, -2.0017) (36.6955, -2.0017) knots 0 0 0 0 1 1 1 1
  line L396 (37.5168, -2.0619) -> (37.3708, -2.0218) construction
  line L397 (37.3708, -2.0218) -> (37.097, -2.0017) construction
  line L398 (37.097, -2.0017) -> (36.6955, -2.0017) construction
  line L399 (35.6608, -2.0017) -> (35.6608, -3.9069)
  line L400 (35.6608, -3.9069) -> (36.7339, -3.9069)
  line L401 (36.6955, -2.0017) -> (35.6608, -2.0017)
  spline S87 degree 3 poles (45.3129, -3.5675) (45.2874, -2.5127) (44.8768, -1.9853) (44.0811, -1.9853) knots 0 0 0 0 1 1 1 1
  line L402 (45.3129, -3.5675) -> (45.2874, -2.5127) construction
  line L403 (45.2874, -2.5127) -> (44.8768, -1.9853) construction
  line L404 (44.8768, -1.9853) -> (44.0811, -1.9853) construction
  spline S88 degree 3 poles (44.0811, -1.9853) (43.1686, -1.9853) (42.7124, -2.7974) (42.7124, -4.4216) knots 0 0 0 0 1 1 1 1
  line L405 (44.0811, -1.9853) -> (43.1686, -1.9853) construction
  line L406 (43.1686, -1.9853) -> (42.7124, -2.7974) construction
  line L407 (42.7124, -2.7974) -> (42.7124, -4.4216) construction
  spline S89 degree 3 poles (42.7124, -4.4216) (42.7124, -5.3596) (42.8365, -5.9965) (43.0847, -6.3323) knots 0 0 0 0 1 1 1 1
  line L408 (42.7124, -4.4216) -> (42.7124, -5.3596) construction
  line L409 (42.7124, -5.3596) -> (42.8365, -5.9965) construction
  line L410 (42.8365, -5.9965) -> (43.0847, -6.3323) construction
  spline S90 degree 3 poles (43.0847, -6.3323) (43.3329, -6.6644) (43.6796, -6.8305) (44.1249, -6.8305) knots 0 0 0 0 1 1 1 1
  line L411 (43.0847, -6.3323) -> (43.3329, -6.6644) construction
  line L412 (43.3329, -6.6644) -> (43.6796, -6.8305) construction
  line L413 (43.6796, -6.8305) -> (44.1249, -6.8305) construction
  spline S91 degree 3 poles (44.1249, -6.8305) (44.8476, -6.8305) (45.2892, -6.3597) (45.4498, -5.418) knots 0 0 0 0 1 1 1 1
  line L414 (44.1249, -6.8305) -> (44.8476, -6.8305) construction
  line L415 (44.8476, -6.8305) -> (45.2892, -6.3597) construction
  line L416 (45.2892, -6.3597) -> (45.4498, -5.418) construction
  line L417 (47.147, -3.4525) -> (45.3129, -3.5675)
  spline S92 degree 3 poles (47.147, -5.522) (47.0375, -6.4162) (46.7036, -7.0969) (46.1451, -7.5641) knots 0 0 0 0 1 1 1 1
  line L418 (47.147, -5.522) -> (47.0375, -6.4162) construction
  line L419 (47.0375, -6.4162) -> (46.7036, -7.0969) construction
  line L420 (46.7036, -7.0969) -> (46.1451, -7.5641) construction
  spline S93 degree 3 poles (46.1451, -7.5641) (45.5903, -8.0277) (44.9096, -8.2594) (44.103, -8.2594) knots 0 0 0 0 1 1 1 1
  line L421 (46.1451, -7.5641) -> (45.5903, -8.0277) construction
  line L422 (45.5903, -8.0277) -> (44.9096, -8.2594) construction
  line L423 (44.9096, -8.2594) -> (44.103, -8.2594) construction
  spline S94 degree 3 poles (44.103, -8.2594) (43.1139, -8.2594) (42.3091, -7.9182) (41.6886, -7.2356) knots 0 0 0 0 1 1 1 1
  line L424 (44.103, -8.2594) -> (43.1139, -8.2594) construction
  line L425 (43.1139, -8.2594) -> (42.3091, -7.9182) construction
  line L426 (42.3091, -7.9182) -> (41.6886, -7.2356) construction
  spline S95 degree 3 poles (41.6886, -7.2356) (41.0718, -6.5531) (40.7633, -5.6096) (40.7633, -4.4051) knots 0 0 0 0 1 1 1 1
  line L427 (41.6886, -7.2356) -> (41.0718, -6.5531) construction
  line L428 (41.0718, -6.5531) -> (40.7633, -5.6096) construction
  line L429 (40.7633, -5.6096) -> (40.7633, -4.4051) construction
  spline S96 degree 3 poles (40.7633, -4.4051) (40.7633, -3.2773) (41.0626, -2.3539) (41.6612, -1.6349) knots 0 0 0 0 1 1 1 1
  line L430 (40.7633, -4.4051) -> (40.7633, -3.2773) construction
  line L431 (40.7633, -3.2773) -> (41.0626, -2.3539) construction
  line L432 (41.0626, -2.3539) -> (41.6612, -1.6349) construction
  spline S97 degree 3 poles (41.6612, -1.6349) (42.2598, -0.9158) (43.0774, -0.5563) (44.114, -0.5563) knots 0 0 0 0 1 1 1 1
  line L433 (41.6612, -1.6349) -> (42.2598, -0.9158) construction
  line L434 (42.2598, -0.9158) -> (43.0774, -0.5563) construction
  line L435 (43.0774, -0.5563) -> (44.114, -0.5563) construction
  spline S98 degree 3 poles (44.114, -0.5563) (45.9097, -0.5563) (46.9207, -1.5217) (47.147, -3.4525) knots 0 0 0 0 1 1 1 1
  line L436 (44.114, -0.5563) -> (45.9097, -0.5563) construction
  line L437 (45.9097, -0.5563) -> (46.9207, -1.5217) construction
  line L438 (46.9207, -1.5217) -> (47.147, -3.4525) construction
  line L439 (45.4498, -5.418) -> (47.147, -5.522)
  line L440 (53.9304, -0.6713) -> (53.9304, -8.1445)
  line L441 (53.9304, -8.1445) -> (52.2113, -8.1445)
  line L442 (52.2113, -8.1445) -> (52.2113, -5.0621)
  line L443 (52.2113, -5.0621) -> (49.8735, -5.0621)
  line L444 (49.8735, -5.0621) -> (49.8735, -8.1445)
  line L445 (49.8735, -8.1445) -> (48.1544, -8.1445)
  line L446 (48.1544, -8.1445) -> (48.1544, -0.6713)
  line L447 (48.1544, -0.6713) -> (49.8735, -0.6713)
  line L448 (49.8735, -0.6713) -> (49.8735, -3.5839)
  line L449 (49.8735, -3.5839) -> (52.2113, -3.5839)
  line L450 (52.2113, -3.5839) -> (52.2113, -0.6713)
  line L451 (52.2113, -0.6713) -> (53.9304, -0.6713)
  line L452 (-61.9705, 20.7969) -> (-8.4036, 20.7969) construction
  line L453 (-8.4036, 20.7969) -> (-8.4036, -16.9712) construction
  line L454 (-8.4036, -16.9712) -> (-61.9705, -16.9712) construction
  line L455 (-61.9705, -16.9712) -> (-61.9705, 20.7969) construction
  line L456 (-43.6246, 13.0785) -> (-43.6246, 19.0282)
  line L457 (-43.6246, 19.0282) -> (-42.4127, 19.0282)
  line L458 (-42.4127, 19.0282) -> (-42.4127, 14.0937)
  line L459 (-42.4127, 14.0937) -> (-39.3989, 14.0937)
  line L460 (-39.3989, 14.0937) -> (-39.3989, 13.0785)
  line L461 (-39.3989, 13.0785) -> (-43.6246, 13.0785)
  spline S99 degree 2 poles (-38.7816, 16.0419) (-38.7816, 16.9565) (-38.5072, 17.5785) knots 0 0 0 1 1 1
  spline S100 degree 2 poles (-38.5072, 17.5785) (-38.3014, 18.0358) (-37.5925, 18.7675) (-37.1718, 18.9413) knots 0 0 0 1 2 2 2
  spline S101 degree 2 poles (-37.1718, 18.9413) (-36.6139, 19.1791) (-35.8776, 19.1791) knots 0 0 0 1 1 1
  spline S102 degree 2 poles (-35.8776, 19.1791) (-34.5514, 19.1791) (-32.9599, 17.5327) (-32.9599, 16.0693) knots 0 0 0 1 2 2 2
  spline S103 degree 2 poles (-32.9599, 16.0693) (-32.9599, 14.6196) (-34.5422, 12.9778) (-35.8639, 12.9778) knots 0 0 0 1 2 2 2
  spline S104 degree 2 poles (-35.8639, 12.9778) (-37.1993, 12.9778) (-38.7816, 14.6105) (-38.7816, 16.0419) knots 0 0 0 1 2 2 2
  spline S105 degree 2 poles (-37.5331, 16.083) (-37.5331, 15.0632) (-36.591, 14.0114) (-35.8639, 14.0114) knots 0 0 0 1 2 2 2
  spline S106 degree 2 poles (-35.8639, 14.0114) (-35.1368, 14.0114) (-34.2084, 15.0541) (-34.2084, 16.0968) knots 0 0 0 1 2 2 2
  spline S107 degree 2 poles (-34.2084, 16.0968) (-34.2084, 17.1303) (-35.1139, 18.1455) (-35.8639, 18.1455) knots 0 0 0 1 2 2 2
  spline S108 degree 2 poles (-35.8639, 18.1455) (-36.6139, 18.1455) (-37.5331, 17.1166) (-37.5331, 16.083) knots 0 0 0 1 2 2 2
  line L462 (-29.2236, 15.2782) -> (-29.2236, 16.2934)
  line L463 (-29.2236, 16.2934) -> (-26.6124, 16.2934)
  line L464 (-26.6124, 16.2934) -> (-26.6124, 13.9062)
  spline S109 degree 2 poles (-26.6124, 13.9062) (-26.9919, 13.5358) (-28.4371, 12.9778) (-29.1779, 12.9778) knots 0 0 0 1 2 2 2
  spline S110 degree 2 poles (-29.1779, 12.9778) (-30.12, 12.9778) (-31.5194, 13.769) (-32.2236, 15.237) (-32.2236, 16.0968) knots 0 0 0 1 2 3 3 3
  spline S111 degree 2 poles (-32.2236, 16.0968) (-32.2236, 17.0343) (-31.4371, 18.4931) (-30.6825, 18.8818) knots 0 0 0 1 2 2 2
  spline S112 degree 2 poles (-30.6825, 18.8818) (-30.1017, 19.1791) (-29.2419, 19.1791) knots 0 0 0 1 1 1
  spline S113 degree 2 poles (-29.2419, 19.1791) (-28.1261, 19.1791) (-26.8685, 18.2416) (-26.6901, 17.4138) knots 0 0 0 1 2 2 2
  line L465 (-26.6901, 17.4138) -> (-27.8929, 17.1897)
  spline S114 degree 2 poles (-27.8929, 17.1897) (-28.0209, 17.6333) (-28.7206, 18.1455) (-29.2419, 18.1455) knots 0 0 0 1 2 2 2
  spline S115 degree 2 poles (-29.2419, 18.1455) (-30.0377, 18.1455) (-30.9752, 17.1394) (-30.9752, 16.1471) knots 0 0 0 1 2 2 2
  spline S116 degree 2 poles (-30.9752, 16.1471) (-30.9752, 15.0815) (-30.0239, 14.0114) (-29.2557, 14.0114) knots 0 0 0 1 2 2 2
  spline S117 degree 2 poles (-29.2557, 14.0114) (-28.8761, 14.0114) (-28.1124, 14.3086) (-27.838, 14.519) knots 0 0 0 1 2 2 2
  line L466 (-27.838, 14.519) -> (-27.838, 15.2782)
  line L467 (-27.838, 15.2782) -> (-29.2236, 15.2782)
  line L468 (-54.838, 3.6362) -> (-54.838, 9.6362)
  line L469 (-54.838, 9.6362) -> (-52.8944, 9.6362)
  spline S118 degree 2 poles (-52.8944, 9.6362) (-51.7877, 9.6362) (-51.4538, 9.5448) knots 0 0 0 1 1 1
  spline S119 degree 2 poles (-51.4538, 9.5448) (-50.9371, 9.4122) (-50.2419, 8.5067) (-50.2419, 7.7887) knots 0 0 0 1 2 2 2
  spline S120 degree 2 poles (-50.2419, 7.7887) (-50.2419, 7.2399) (-50.6444, 6.4853) (-51.2618, 6.0555) (-51.5819, 5.9869) knots 0 0 0 1 2 3 3 3
  spline S121 degree 2 poles (-51.5819, 5.9869) (-52.0118, 5.9) (-52.8349, 5.9) knots 0 0 0 1 1 1
  line L470 (-52.8349, 5.9) -> (-53.6261, 5.9)
  line L471 (-53.6261, 5.9) -> (-53.6261, 3.6362)
  line L472 (-53.6261, 3.6362) -> (-54.838, 3.6362)
  line L473 (-53.6261, 8.621) -> (-53.6261, 6.9152)
  line L474 (-53.6261, 6.9152) -> (-52.963, 6.9152)
  spline S122 degree 2 poles (-52.963, 6.9152) (-52.245, 6.9152) (-51.7648, 7.1027) (-51.4904, 7.5051) (-51.4904, 7.7704) knots 0 0 0 1 2 3 3 3
  spline S123 degree 2 poles (-51.4904, 7.7704) (-51.4904, 8.0997) (-51.8746, 8.525) (-52.1718, 8.5798) knots 0 0 0 1 2 2 2
  spline S124 degree 2 poles (-52.1718, 8.5798) (-52.3868, 8.621) (-53.0407, 8.621) knots 0 0 0 1 1 1
  line L475 (-53.0407, 8.621) -> (-53.6261, 8.621)
  line L476 (-49.245, 3.6362) -> (-49.245, 9.6362)
  line L477 (-49.245, 9.6362) -> (-44.7953, 9.6362)
  line L478 (-44.7953, 9.6362) -> (-44.7953, 8.621)
  line L479 (-44.7953, 8.621) -> (-48.0331, 8.621)
  line L480 (-48.0331, 8.621) -> (-48.0331, 7.2902)
  line L481 (-48.0331, 7.2902) -> (-45.0194, 7.2902)
  line L482 (-45.0194, 7.2902) -> (-45.0194, 6.275)
  line L483 (-45.0194, 6.275) -> (-48.0331, 6.275)
  line L484 (-48.0331, 6.275) -> (-48.0331, 4.6515)
  line L485 (-48.0331, 4.6515) -> (-44.681, 4.6515)
  line L486 (-44.681, 4.6515) -> (-44.681, 3.6362)
  line L487 (-44.681, 3.6362) -> (-49.245, 3.6362)
  line L488 (-43.652, 3.6362) -> (-43.652, 9.6362)
  line L489 (-43.652, 9.6362) -> (-41.1002, 9.6362)
  spline S125 degree 2 poles (-41.1002, 9.6362) (-40.1352, 9.6362) (-39.2663, 9.3115) (-38.7404, 8.4884) (-38.7404, 7.9533) knots 0 0 0 1 2 3 3 3
  spline S126 degree 2 poles (-38.7404, 7.9533) (-38.7404, 7.2811) (-39.5316, 6.3984) (-40.3227, 6.2841) knots 0 0 0 1 2 2 2
  spline S127 degree 2 poles (-40.3227, 6.2841) (-39.9294, 6.0555) (-39.4172, 5.5067) (-38.9828, 4.807) knots 0 0 0 1 2 2 2
  line L490 (-38.9828, 4.807) -> (-38.2511, 3.6362)
  line L491 (-38.2511, 3.6362) -> (-39.7008, 3.6362)
  line L492 (-39.7008, 3.6362) -> (-40.5743, 4.9442)
  spline S128 degree 2 poles (-40.5743, 4.9442) (-41.0453, 5.6439) (-41.3883, 6.0097) (-41.7724, 6.1423) (-42.1932, 6.1423) knots 0 0 0 1 2 3 3 3
  line L493 (-42.1932, 6.1423) -> (-42.4401, 6.1423)
  line L494 (-42.4401, 6.1423) -> (-42.4401, 3.6362)
  line L495 (-42.4401, 3.6362) -> (-43.652, 3.6362)
  line L496 (-42.4401, 7.0981) -> (-41.5438, 7.0981)
  spline S129 degree 2 poles (-41.5438, 7.0981) (-40.6703, 7.0981) (-40.2358, 7.2445) (-39.9889, 7.6058) (-39.9889, 7.8756) knots 0 0 0 1 2 3 3 3
  spline S130 degree 2 poles (-39.9889, 7.8756) (-39.9889, 8.1774) (-40.3136, 8.5524) (-40.6063, 8.6027) knots 0 0 0 1 2 2 2
  spline S131 degree 2 poles (-40.6063, 8.6027) (-40.7572, 8.621) (-41.4935, 8.621) knots 0 0 0 1 1 1
  line L497 (-41.4935, 8.621) -> (-42.4401, 8.621)
  line L498 (-42.4401, 8.621) -> (-42.4401, 7.0981)
  line L499 (-37.6383, 3.6362) -> (-37.6383, 9.6362)
  line L500 (-37.6383, 9.6362) -> (-36.4264, 9.6362)
  line L501 (-36.4264, 9.6362) -> (-36.4264, 3.6362)
  line L502 (-36.4264, 3.6362) -> (-37.6383, 3.6362)
  spline S132 degree 2 poles (-35.5163, 6.5997) (-35.5163, 7.5143) (-35.2419, 8.1362) knots 0 0 0 1 1 1
  spline S133 degree 2 poles (-35.2419, 8.1362) (-35.0361, 8.5936) (-34.3273, 9.3253) (-33.9066, 9.499) knots 0 0 0 1 2 2 2
  spline S134 degree 2 poles (-33.9066, 9.499) (-33.3486, 9.7369) (-32.6124, 9.7369) knots 0 0 0 1 1 1
  spline S135 degree 2 poles (-32.6124, 9.7369) (-31.2861, 9.7369) (-29.6947, 8.0905) (-29.6947, 6.6271) knots 0 0 0 1 2 2 2
  spline S136 degree 2 poles (-29.6947, 6.6271) (-29.6947, 5.1774) (-31.277, 3.5356) (-32.5986, 3.5356) knots 0 0 0 1 2 2 2
  spline S137 degree 2 poles (-32.5986, 3.5356) (-33.934, 3.5356) (-35.5163, 5.1683) (-35.5163, 6.5997) knots 0 0 0 1 2 2 2
  spline S138 degree 2 poles (-34.2679, 6.6408) (-34.2679, 5.621) (-33.3258, 4.5692) (-32.5986, 4.5692) knots 0 0 0 1 2 2 2
  spline S139 degree 2 poles (-32.5986, 4.5692) (-31.8715, 4.5692) (-30.9432, 5.6119) (-30.9432, 6.6545) knots 0 0 0 1 2 2 2
  spline S140 degree 2 poles (-30.9432, 6.6545) (-30.9432, 7.6881) (-31.8486, 8.7033) (-32.5986, 8.7033) knots 0 0 0 1 2 2 2
  spline S141 degree 2 poles (-32.5986, 8.7033) (-33.3486, 8.7033) (-34.2679, 7.6744) (-34.2679, 6.6408) knots 0 0 0 1 2 2 2
  line L503 (-28.7572, 9.6362) -> (-26.5392, 9.6362)
  spline S142 degree 2 poles (-26.5392, 9.6362) (-25.7892, 9.6362) (-25.3959, 9.5219) knots 0 0 0 1 1 1
  spline S143 degree 2 poles (-25.3959, 9.5219) (-24.87, 9.3664) (-24.1154, 8.5707) (-23.7221, 7.4228) (-23.7221, 6.5768) knots 0 0 0 1 2 3 3 3
  spline S144 degree 2 poles (-23.7221, 6.5768) (-23.7221, 5.8359) (-23.905, 5.3009) knots 0 0 0 1 1 1
  spline S145 degree 2 poles (-23.905, 5.3009) (-24.1337, 4.6469) (-24.5499, 4.2399) knots 0 0 0 1 1 1
  spline S146 degree 2 poles (-24.5499, 4.2399) (-24.8654, 3.9335) (-25.4005, 3.7643) knots 0 0 0 1 1 1
  spline S147 degree 2 poles (-25.4005, 3.7643) (-25.8029, 3.6362) (-26.4752, 3.6362) knots 0 0 0 1 1 1
  line L504 (-26.4752, 3.6362) -> (-28.7572, 3.6362)
  line L505 (-28.7572, 3.6362) -> (-28.7572, 9.6362)
  line L506 (-27.5453, 8.621) -> (-27.5453, 4.6515)
  line L507 (-27.5453, 4.6515) -> (-26.6398, 4.6515)
  spline S148 degree 2 poles (-26.6398, 4.6515) (-26.1276, 4.6515) (-25.9035, 4.7109) knots 0 0 0 1 1 1
  spline S149 degree 2 poles (-25.9035, 4.7109) (-25.6063, 4.7841) (-25.2175, 5.1317) (-24.9706, 5.9411) (-24.9706, 6.6362) knots 0 0 0 1 2 3 3 3
  spline S150 degree 2 poles (-24.9706, 6.6362) (-24.9706, 7.3314) (-25.2175, 8.0722) (-25.6611, 8.4884) (-25.9996, 8.5615) knots 0 0 0 1 2 3 3 3
  spline S151 degree 2 poles (-25.9996, 8.5615) (-26.2557, 8.621) (-27.0011, 8.621) knots 0 0 0 1 1 1
  line L508 (-27.0011, 8.621) -> (-27.5453, 8.621)
  line L509 (-22.7343, 3.6362) -> (-22.7343, 9.6362)
  line L510 (-22.7343, 9.6362) -> (-21.5224, 9.6362)
  line L511 (-21.5224, 9.6362) -> (-21.5224, 3.6362)
  line L512 (-21.5224, 3.6362) -> (-22.7343, 3.6362)
  line L513 (-16.5285, 5.8451) -> (-15.3532, 5.4747)
  spline S152 degree 2 poles (-15.3532, 5.4747) (-15.623, 4.4914) (-16.8807, 3.5356) (-17.8456, 3.5356) knots 0 0 0 1 2 2 2
  spline S153 degree 2 poles (-17.8456, 3.5356) (-19.0392, 3.5356) (-20.5804, 5.1683) (-20.5804, 6.5814) knots 0 0 0 1 2 2 2
  spline S154 degree 2 poles (-20.5804, 6.5814) (-20.5804, 8.0814) (-19.0346, 9.7369) (-17.7724, 9.7369) knots 0 0 0 1 2 2 2